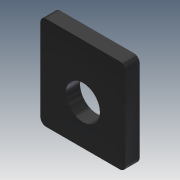
# Autodesk Inventor part: HbSensorCushion01
Saved by Autodesk Inventor 2015 SP1 (Build 190203100, 203)
## iProperties
Created: 2015-05-23
Part Number: HbSensorCushion01
Material: ゴム
Document SubType Name: Modeling
Designer: Yamaura
Density: 0.93 g/cm^3
Appearance: ゴム - 黒 - バージョン 1.1
Author: Yamaura
Autodesk Inventor part; units mm, degrees
ref_plane "YZ Plane" through (0, 0, 0) normal (1, 0, 0) x (0, 1, 0)
ref_plane "XZ Plane" through (0, 0, 0) normal (0, 1, 0) x (-1, 0, 0)
ref_plane "XY Plane" through (0, 0, 0) normal (0, 0, 1) x (1, 0, 0)
sketch "スケッチ1" plane through (0, 0, 0) normal (0, 0, 1) x (1, 0, 0)
  line L0 (-15, 19.05) -> (15, 19.05)
  line L1 (15, 19.05) -> (15, -13.95)
  line L2 (15, -13.95) -> (-15, -13.95)
  line L3 (-15, -13.95) -> (-15, 19.05)
  point P0 (0, 0)
  dimension "d0" = 30
  dimension "d1" = 33
  dimension "d2" = 19.05
  dimension "d3" = 15
  constraints: 8 end point, 2 parallel, 1 horizontal, 1 perpendicular
  measures "d0" distance of L0.start L0.end
  measures "d1" distance of L2.end L0.start
  measures "d2" distance from line of point (0, 0) L0
  measures "d3" distance from line of L1 point (0, 0)
extrude "押し出し1" add sketch "スケッチ1" along normal blind 5
sketch "スケッチ2" plane through (0, 0, 0) normal (0, 0, 1) x (1, 0, 0)
  circle A0 centre (0, 0) radius 6
  dimension "d6" = 12
  constraints: 1 centre point, 1 coincident
  measures "d6" diameter of A0
extrude "押し出し2" cut sketch "スケッチ2" along normal blind 5
fillet "フィレット1" radius 2 4 edges at (15, 19.05, 2.5) (15, -13.95, 2.5) (-15, -13.95, 2.5) (-15, 19.05, 2.5)
